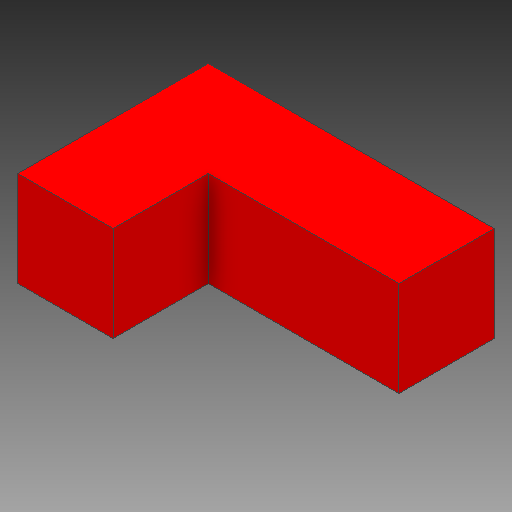
# Autodesk Inventor part: Red part
Saved by Autodesk Inventor 2017 (Build 210142000, 142)
## iProperties
Created: 2016-11-01
Part Number: Red part
Material: Generic
Document SubType Name: Modeling
Designer: rbibb
Density: 1 g/cm^3
Appearance: Default
Mass: 27.6532 g
Surface Area: 65.3224 cm^2
Volume: 27.6532 cm^3
Author: rbibb
Autodesk Inventor part; units mm, degrees
ref_plane "YZ Plane" through (0, 0, 0) normal (1, 0, 0) x (0, 1, 0)
ref_plane "XZ Plane" through (0, 0, 0) normal (0, 1, 0) x (-1, 0, 0)
ref_plane "XY Plane" through (0, 0, 0) normal (0, 0, 1) x (1, 0, 0)
sketch "Sketch1" plane through (0, 0, 0) normal (1, 0, 0) x (0, 1, 0)
  line L0 (13.1786, 29.8851) -> (-5.8714, 29.8851)
  line L1 (-5.8714, 29.8851) -> (-5.8714, -27.2649)
  line L2 (-5.8714, -27.2649) -> (13.1786, -27.2649)
  line L3 (13.1786, -27.2649) -> (13.1786, 29.8851)
  point P0 (0, 0)
  dimension "d0" = 19.05
  dimension "d1" = 57.15
  constraints: 8 end point, 2 parallel, 1 horizontal, 1 perpendicular
  measures "d0" distance of L2.end L1.end
  measures "d1" distance of L1.end L0.end
extrude "Extrusion1" add sketch "Sketch1" along normal blind 19.05
sketch "Sketch2" plane through (19.05, 0, 0) normal (1, 0, 0) x (0, 0, -1)
  line L0 (-29.8851, 13.1786) -> (-29.8851, -5.8714) projected
  line L1 (27.2649, 13.1786) -> (-29.8851, 13.1786) projected
  line L2 (-29.8851, -5.8714) -> (-10.8351, -5.8714)
  line L3 (-10.8351, -5.8714) -> (-10.8351, 13.1786)
  line L4 (-10.8351, 13.1786) -> (-29.8851, 13.1786)
  line L5 (-29.8851, 13.1786) -> (-29.8851, -5.8714)
  point P0 (0, 0)
  dimension "d4" = 19.05
  constraints: 8 end point, 2 parallel, 1 horizontal, 1 perpendicular, 1 point on line
  measures "d4" distance of L4.end L3.end
extrude "Extrusion2" add sketch "Sketch2" along normal blind 19.05
body "Solid1"
